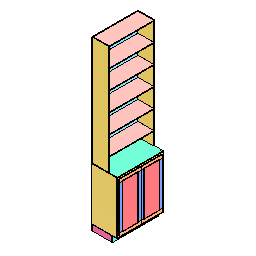
MS_BookShelves (Autodesk Fusion 360 design; units mm, degrees)
Autodesk Fusion 360 part; units mm, degrees
sketch "Part List" plane through (0, 0, 0) normal (1, 0, 0) x (0, 1, 0)
  line L0 (-117.4604, 5.2821) -> (-27.4764, 5.2821) construction
  line L1 (-27.4764, 5.2821) -> (-27.4764, 106.5384) construction
  line L2 (-27.4764, 106.5384) -> (-117.4604, 106.5384) construction
  line L3 (-117.4604, 106.5384) -> (-117.4604, 5.2821) construction
  dimension "d1" = 2
sketch "Room" plane through (0, 0, 0) normal (0, 0, 1) x (1, 0, 0)
  line L0 (922.3375, 3178.175) -> (2225.675, 3178.175) construction
  line L1 (0, 3178.175) -> (922.3375, 3178.175) construction
  line L2 (2225.675, 3178.175) -> (3114.675, 3178.175) construction
  line L3 (2259.0125, 0) -> (1363.6625, 0) construction
  line L4 (1363.6625, 46.449) -> (2259.0125, 46.449) construction
  line L5 (3114.675, 3178.175) -> (3630.6125, 3178.175) construction
  line L6 (0, 0) -> (0, 3178.175) construction
  line L7 (1363.6625, 0) -> (1363.6625, 46.449) construction
  line L8 (58.5758, 2317.75) -> (0, 2317.75) construction
  line L9 (0, 2403.475) -> (58.5758, 2403.475) construction
  line L10 (58.5758, 2403.475) -> (58.5758, 2317.75) construction
  line L11 (140.5097, 3178.175) -> (140.5097, 2420.9375) construction
  line L12 (0, 2317.75) -> (0, 2403.475) construction
  line L13 (0, 0) -> (3648.075, 0) construction
  line L14 (2259.0125, 46.449) -> (2259.0125, 0) construction
  point P0 (0, 2403.475)
  point P1 (0, 2317.75)
  point P2 (2259.0125, 0)
  point P3 (1363.6625, 0)
  dimension "d2" = 3648.075
  dimension "d3" = 895.35
  dimension "d4" = 1363.6625
  dimension "d5" = 1389.0625
  dimension "d6" = 3178.175
  dimension "d7" = 922.3375
  dimension "d8" = 1303.3375
  dimension "d9" = 889
  dimension "d10" = 515.9375
  dimension "d11" = 3630.6125
  dimension "d12" = 774.7
  dimension "d13" = 85.725
  dimension "d14" = 757.2375
  dimension "d15" = 90
  constraint coincident L6.start L13.start
  constraint horizontal L13
  constraint coincident P3 L13
  constraint coincident P2 L13
  constraint horizontal L3
  constraint vertical L7
  constraint horizontal L4
  constraint vertical L14
  constraint coincident P2 L3.start
  constraint perpendicular L6 L13
  constraint perpendicular L1 L6
  constraint parallel L0 L1
  constraint parallel L0 L2
  constraint parallel L2 L5
  constraint coincident P0 L6
  constraint coincident P1 L6
  constraint horizontal L9
  constraint vertical L10
  constraint horizontal L8
  constraint vertical L12
  constraint coincident P0 L9.start
  constraint coincident L11.start L1
  constraint perpendicular L1 L11
  measures "d2" distance of L13.end L6.start
  measures "d3" distance of P2 P3
  measures "d4" distance of L6.start P3
  measures "d5" distance of L13.end P2
  measures "d6" distance of L6.start L1.start
  measures "d7" distance of L1.start L0.start
  measures "d8" distance of L0.start L0.end
  measures "d9" distance of L0.end L2.end
  measures "d10" distance of L2.end L5.end
  measures "d11" distance of L1.start L5.end
  measures "d12" distance of L1.start P0
  measures "d13" distance of P0 P1
  measures "d14" distance of L11.start L11.end
  measures "d15" angle of L1 L11
sketch "Celing" plane through (0, 0, 0) normal (0, 0, 1) x (1, 0, 0)
  line L0 (0, 0, 2743.2) -> (3648.075, 0, 2743.2)
  line L1 (3648.075, 0, 2743.2) -> (3648.075, 3178.175, 2743.2)
  line L2 (3648.075, 3178.175, 2743.2) -> (0, 3178.175, 2743.2)
  line L3 (0, 3178.175, 2743.2) -> (0, 0, 2743.2)
  dimension "height" = 2743.2
  dimension "width" = 3648.075
  dimension "length" = 3178.175
ref_plane "WorkPlane1" through (0, 0, 0) normal (0, 1, 0) x (0, 0, 1) in component ">>WSSi_Sides"
sketch "Sketch1" plane through (0, 0, 0) normal (0, 1, 0) x (1, 0, 0) in component ">>WSSi_Sides"
  line L0 (6.35, 0) -> (266.7, 0)
  line L1 (266.7, 0) -> (266.7, -1739.9)
  line L2 (266.7, -1739.9) -> (6.35, -1739.9)
  line L3 (6.35, -1739.9) -> (6.35, 0)
  point P0 (6.35, 0)
  dimension "Y_WSSi_Sides_Orig" = 0
  dimension "X_WSSi_Sides_Orig" = 6.35
  dimension "WSSi_Sides_Width" = 260.35
  dimension "WSSi_Sides_Length" = 1739.9
  constraint horizontal L0
  constraint vertical L1
  constraint horizontal L2
  constraint vertical L3
  constraint coincident P0 L0.start
  measures "Y_WSSi_Sides_Orig" vertical distance of origin L0.start
  measures "X_WSSi_Sides_Orig" horizontal distance of origin L0.start
  measures "WSSi_Sides_Width" distance of P0 L0.end
  measures "WSSi_Sides_Length" distance of P0 L2.end
extrude "Extrude1" add sketch "Sketch1" along normal blind 12.7 makes body 1 in component ">>WSSi_Sides"
pattern_linear "00000000-0000-0000-0000-000000000000" [suppressed] in component "~~~>WS - Sides"
ref_plane "WorkPlane1" through (0, 0, 0) normal (1, 0, 0) x (0, 1, 0) in component ">WS - Back"
sketch "Sketch1 (2)" plane through (0, 0, 0) normal (1, 0, 0) x (0, 1, 0) in component ">WS - Back"
  line L0 (0, 0) -> (736.6, 0)
  line L1 (736.6, 0) -> (736.6, 1739.9)
  line L2 (736.6, 1739.9) -> (0, 1739.9)
  line L3 (0, 1739.9) -> (0, 0)
  line L4 (12.7, 0) -> (723.9, 0)
  line L5 (723.9, 0) -> (723.9, 1727.2)
  line L6 (723.9, 1727.2) -> (12.7, 1727.2)
  line L7 (12.7, 1727.2) -> (12.7, 0)
  point P0 (12.7, 0)
  dimension "WS_Back_Width" = 736.6
  dimension "WS_Back_Length" = 1739.9
  dimension "Y_WS_Back_Orig" = 0
  dimension "X_WS_Back_Orig" = 0
  dimension "WS_Back_Rabbit_Width" = 12.7
  dimension "WS_Back_NoRabbitWidth" = 711.2
  dimension "WS_Back_NoRabbit_Length" = 1727.2
  constraint horizontal L0
  constraint vertical L1
  constraint horizontal L2
  constraint vertical L3
  constraint coincident L0 P0
  constraint horizontal L4
  constraint vertical L5
  constraint horizontal L6
  constraint vertical L7
  constraint coincident P0 L4.start
  measures "WS_Back_Width" distance of L0.start L0.end
  measures "WS_Back_Length" distance of L0.start L2.end
  measures "Y_WS_Back_Orig" vertical distance of L0.start L3.end
  measures "X_WS_Back_Orig" horizontal distance of L0.start L3.end
  measures "WS_Back_Rabbit_Width" distance of L0.start L4.start
  measures "WS_Back_NoRabbitWidth" distance of P0 L4.end
  measures "WS_Back_NoRabbit_Length" distance of P0 L6.end
extrude "Extrude1'" add sketch "Sketch1 (2)" along normal blind 12.7 separate body contours L0 L4 L5 L6 L7 makes body 2 in component ">WS - Back"
extrude "Extrude2" add sketch "Sketch1 (2)" along normal blind 6.35 contours L0 L1 L2 L3 L5 L6 L7 bodies 2 in component ">WS - Back"
ref_plane "WorkPlane1" through (12.7, 0, 0) normal (1, 0, 0) x (0, 1, 0) in component "WSS_Shelves_"
sketch "Sketch1 (3)" plane through (12.7, 0, 0) normal (1, 0, 0) x (0, 1, 0) in component "WSS_Shelves_"
  line L0 (12.7, 1727.2) -> (723.9, 1727.2)
  line L1 (12.7, 1739.9) -> (12.7, 1727.2)
  line L2 (723.9, 1739.9) -> (12.7, 1739.9)
  line L3 (723.9, 1727.2) -> (723.9, 1739.9)
  point P0 (12.7, 1727.2)
  dimension "WSS_Shelves_Length" = 711.2
  dimension "WSS_Shelves_Thickness" = 12.7
  dimension "Y_WSS_Shelves_Orig" = 12.7
  dimension "Z_WSS_Shelves_Orig" = 1727.2
  constraint horizontal L0
  constraint vertical L3
  constraint horizontal L2
  constraint vertical L1
  constraint coincident P0 L0.start
  measures "WSS_Shelves_Length" distance of P0 L0.end
  measures "WSS_Shelves_Thickness" distance of P0 L1.start
  measures "Y_WSS_Shelves_Orig" horizontal distance of origin P0
  measures "Z_WSS_Shelves_Orig" vertical distance of origin P0
extrude "Extrude1''" add sketch "Sketch1 (3)" along normal blind 254 separate body makes body 3 in component "WSS_Shelves_"
pattern_linear "00000000-0000-0000-0000-000000000000'" [suppressed] in component "~~~>WS - Shelves"
ref_plane "WorkPlane1" through (266.7, 0, 0) normal (1, 0, 0) x (0, 1, 0) in component "~~~>WS - Molding"
sketch "Sketch1 (4)" plane through (266.7, 0, 0) normal (1, 0, 0) x (0, 1, 0) in component "WSM_Molding"
  line L0 (0, 0) -> (38.1, 0)
  line L1 (38.1, 0) -> (38.1, 1739.9)
  line L2 (38.1, 1739.9) -> (0, 1739.9)
  line L3 (0, 1739.9) -> (0, 0)
  dimension "X_WSM_Molding_Orig" = 0
  dimension "Y_WSM_Molding_Orig" = 0
  dimension "WSM_Molding_Width" = 38.1
  dimension "WSM_Molding_Length" = 1739.9
  constraint horizontal L0
  constraint vertical L1
  constraint horizontal L2
  constraint vertical L3
  constraint coincident L0.start L3.end
  measures "X_WSM_Molding_Orig" horizontal distance of L0.start L3.end
  measures "Y_WSM_Molding_Orig" vertical distance of L0.start L3.end
  measures "WSM_Molding_Width" distance of L0.start L0.end
  measures "WSM_Molding_Length" distance of L0.start L2.end
extrude "Extrude1'''" add sketch "Sketch1 (4)" along normal blind 12.7 separate body makes body 4 in component "WSM_Molding"
pattern_linear "00000000-0000-0000-0000-000000000000''" [suppressed] in component "~~~>WS - Molding"
ref_plane "WorkPlane1" through (0, 0, -12.7) normal (0, 0, 1) x (1, 0, 0) in component ">>WCT_TableTop"
sketch "Sketch1 (5)" plane through (0, 0, -12.7) normal (0, 0, 1) x (1, 0, 0) in component ">>WCT_TableTop"
  line L0 (0, 0) -> (406.4, 0)
  line L1 (406.4, 0) -> (406.4, 736.6)
  line L2 (406.4, 736.6) -> (0, 736.6)
  line L3 (0, 736.6) -> (0, 0)
  dimension "Y_WC_TableTop_Orig" = 0
  dimension "X_WC_TableTop_Orig" = 0
  dimension "WCT_TableTop_Width" = 406.4
  dimension "WCT_TableTop_Length" = 736.6
  constraint horizontal L0
  constraint vertical L1
  constraint horizontal L2
  constraint vertical L3
  constraint coincident L0.start L3.end
  measures "Y_WC_TableTop_Orig" horizontal distance of L0.start L3.end
  measures "X_WC_TableTop_Orig" vertical distance of L0.start L3.end
  measures "WCT_TableTop_Width" distance of L0.start L0.end
  measures "WCT_TableTop_Length" distance of L0.start L2.end
extrude "Extrude1''''" add sketch "Sketch1 (5)" along normal blind 12.7 separate body makes body 5 in component ">>WCT_TableTop"
ref_plane "WorkPlane1" through (0, 0, -850.9) normal (0, 0, 1) x (1, 0, 0) in component ">>WCB_Bottom"
sketch "Sketch1 (6)" plane through (0, 0, -850.9) normal (0, 0, 1) x (1, 0, 0) in component ">>WCB_Bottom"
  line L0 (0, 0) -> (406.4, 0)
  line L1 (406.4, 0) -> (406.4, 736.6)
  line L2 (406.4, 736.6) -> (0, 736.6)
  line L3 (0, 736.6) -> (0, 0)
  line L4 (393.7, 12.7) -> (393.7, 723.9)
  line L5 (393.7, 723.9) -> (12.7, 723.9)
  line L6 (12.7, 723.9) -> (12.7, 12.7)
  line L7 (12.7, 12.7) -> (393.7, 12.7)
  dimension "Y_WC_Bottom_Orig" = 0
  dimension "X_WC_Bottom_Orig" = 0
  dimension "WCBo_Bottom_Width" = 406.4
  dimension "WCBo_Bottom_Length" = 736.6
  constraint horizontal L0
  constraint vertical L1
  constraint horizontal L2
  constraint vertical L3
  constraint coincident L0.start L3.end
  measures "Y_WC_Bottom_Orig" vertical distance of L0.start L3.end
  measures "X_WC_Bottom_Orig" horizontal distance of L0.start L3.end
  measures "WCBo_Bottom_Width" distance of L0.start L0.end
  measures "WCBo_Bottom_Length" distance of L0.start L2.end
extrude "Extrude1'''''" add sketch "Sketch1 (6)" along normal blind 12.7 separate body contours L4 L5 L6 L7 makes body 6 in component ">>WCB_Bottom"
extrude "Extrude2'" add sketch "Sketch1 (6)" along normal blind 6.35 bodies 6 in component ">>WCB_Bottom"
ref_plane "WorkPlane1" through (0, 0, 0) normal (0, 1, 0) x (0, 0, 1) in component ">>WCS_Sides"
sketch "Sketch1 (7)" plane through (0, 0, 0) normal (0, 1, 0) x (1, 0, 0) in component ">>WCS_Sides"
  line L0 (0, 844.55) -> (393.7, 844.55)
  line L1 (393.7, 844.55) -> (393.7, 12.7)
  line L2 (393.7, 12.7) -> (0, 12.7)
  line L3 (0, 12.7) -> (0, 844.55)
  point P0 (0, 844.55)
  dimension "X_WC_Sides_Orig" = 0
  dimension "WCS_Sides_Width" = 393.7
  dimension "WCS_Sides_Length" = 831.85
  constraint horizontal L0
  constraint vertical L1
  constraint horizontal L2
  constraint vertical L3
  constraint coincident P0 L0.start
  measures "X_WC_Sides_Orig" horizontal distance of origin L0.start
  measures "WCS_Sides_Width" distance of P0 L0.end
  measures "WCS_Sides_Length" distance of P0 L2.end
extrude "Extrude1''''''" add sketch "Sketch1 (7)" along normal blind 12.7 separate body makes body 7 in component ">>WCS_Sides"
pattern_linear "00000000-0000-0000-0000-000000000000'''" [suppressed] in component "~~~>WC - Sides"
ref_plane "WorkPlane1" through (0, 0, 0) normal (1, 0, 0) x (0, 1, 0) in component ">>WCBa_Back"
sketch "Sketch1 (8)" plane through (0, 0, 0) normal (1, 0, 0) x (0, 1, 0) in component ">>WCBa_Back"
  line L0 (12.7, -844.55) -> (723.9, -844.55)
  line L1 (723.9, -844.55) -> (723.9, -12.7)
  line L2 (723.9, -12.7) -> (12.7, -12.7)
  line L3 (12.7, -12.7) -> (12.7, -844.55)
  point P0 (12.7, -844.55)
  dimension "Y_WC_Back_Orig" = 12.7
  dimension "WCBa_Back_Width" = 711.2
  dimension "WCBa_Back_Length" = 831.85
  constraint horizontal L0
  constraint vertical L1
  constraint horizontal L2
  constraint vertical L3
  constraint coincident P0 L0.start
  measures "Y_WC_Back_Orig" horizontal distance of origin L0.start
  measures "WCBa_Back_Width" distance of P0 L0.end
  measures "WCBa_Back_Length" distance of P0 L2.end
extrude "Extrude1'''''''" add sketch "Sketch1 (8)" along normal blind 12.7 separate body makes body 8 in component ">>WCBa_Back"
ref_plane "WorkPlane1" through (0, 0, -419.1) normal (0, 0, 1) x (1, 0, 0) in component "WCS_Shelves"
sketch "Sketch1 (9)" plane through (0, 0, -419.1) normal (0, 0, 1) x (1, 0, 0) in component "WCS_Shelves"
  line L0 (12.7, 12.7) -> (393.7, 12.7)
  line L1 (393.7, 12.7) -> (393.7, 723.9)
  line L2 (393.7, 723.9) -> (12.7, 723.9)
  line L3 (12.7, 723.9) -> (12.7, 12.7)
  point P0 (12.7, 12.7)
  dimension "Y_WC_Shelves_Orig" = 12.7
  dimension "X_WC_Shelves_Orig" = 12.7
  dimension "WCS_Shelves_Width" = 381
  dimension "WCS_Shelves_Length" = 711.2
  constraint horizontal L0
  constraint vertical L1
  constraint horizontal L2
  constraint vertical L3
  constraint coincident P0 L0.start
  measures "Y_WC_Shelves_Orig" vertical distance of origin L0.start
  measures "X_WC_Shelves_Orig" horizontal distance of origin L0.start
  measures "WCS_Shelves_Width" distance of P0 L0.end
  measures "WCS_Shelves_Length" distance of P0 L2.end
extrude "Extrude1''''''''" add sketch "Sketch1 (9)" along normal blind 12.7 separate body makes body 9 in component "WCS_Shelves"
ref_plane "WorkPlane1" through (393.7, 0, 0) normal (1, 0, 0) x (0, 1, 0) in component ">>WCF - Top/Bottom"
sketch "Sketch1 (10)" plane through (393.7, 0, 0) normal (1, 0, 0) x (0, 1, 0) in component ">>WCF - Top/Bottom"
  line L0 (0, -12.7) -> (736.6, -12.7)
  line L1 (736.6, -12.7) -> (736.6, -50.8)
  line L2 (736.6, -50.8) -> (0, -50.8)
  line L3 (0, -50.8) -> (0, -12.7)
  point P0 (0, -12.7)
  dimension "Y_WCF_TopBottom_Orig" = 0
  dimension "Z_WCF_TopBottom_Orig" = 12.7
  dimension "WCF_TopBottom_Length" = 736.6
  dimension "WCF_TopBottom_Width" = 38.1
  constraint horizontal L0
  constraint vertical L1
  constraint horizontal L2
  constraint vertical L3
  constraint coincident P0 L0.start
  measures "Y_WCF_TopBottom_Orig" horizontal distance of origin L0.start
  measures "Z_WCF_TopBottom_Orig" vertical distance of origin L0.start
  measures "WCF_TopBottom_Length" distance of P0 L0.end
  measures "WCF_TopBottom_Width" distance of P0 L2.end
extrude "Extrude1'''''''''" add sketch "Sketch1 (10)" along normal blind 12.7 separate body makes body 10 in component ">>WCF - Top/Bottom"
pattern_linear "00000000-0000-0000-0000-000000000000''''" [suppressed] in component "~~~>WC - Front"
ref_plane "WorkPlane1" through (393.7, 0, 0) normal (1, 0, 0) x (0, 1, 0) in component ">>WCF - Left/Right"
sketch "Sketch1 (11)" plane through (393.7, 0, 0) normal (1, 0, 0) x (0, 1, 0) in component ">>WCF - Left/Right"
  line L0 (0, -50.8) -> (38.1, -50.8)
  line L1 (38.1, -50.8) -> (38.1, -806.45)
  line L2 (38.1, -806.45) -> (0, -806.45)
  line L3 (0, -806.45) -> (0, -50.8)
  point P0 (0, -50.8)
  dimension "Y_WCF_LeftRight_Orig" = 0
  dimension "Z_WCF_LeftRight_Orig" = 50.8
  dimension "WCF_LeftRight_Width" = 38.1
  dimension "WCF_LeftRight_Length" = 755.65
  constraint horizontal L0
  constraint vertical L1
  constraint horizontal L2
  constraint vertical L3
  constraint coincident P0 L0.start
  measures "Y_WCF_LeftRight_Orig" horizontal distance of origin L0.start
  measures "Z_WCF_LeftRight_Orig" vertical distance of origin L0.start
  measures "WCF_LeftRight_Width" distance of P0 L0.end
  measures "WCF_LeftRight_Length" distance of P0 L2.end
extrude "Extrude1''''''''''" add sketch "Sketch1 (11)" along normal blind 12.7 separate body makes body 11 in component ">>WCF - Left/Right"
pattern_linear "00000000-0000-0000-0000-000000000000'''''" [suppressed] in component "~~~>WC - Front"
ref_plane "WorkPlane1" through (406.4, 0, 0) normal (1, 0, 0) x (0, 1, 0) in component ">>WCD - Top/Bottom"
sketch "Sketch1 (12)" plane through (406.4, 0, 0) normal (1, 0, 0) x (0, 1, 0) in component ">>WCD - Top/Bottom"
  line L0 (25.4, -31.75) -> (366.7125, -31.75)
  line L1 (366.7125, -31.75) -> (366.7125, -82.55)
  line L2 (366.7125, -82.55) -> (25.4, -82.55)
  line L3 (25.4, -82.55) -> (25.4, -31.75)
  point P0 (25.4, -31.75)
  dimension "Y_WCD_TopBottom_Orig" = 25.4
  dimension "Z_WCD_TopBottom_Orig" = 31.75
  dimension "WCD_TopBottom_Length" = 341.3125
  dimension "WCD_TopBottom_Width" = 50.8
  constraint horizontal L0
  constraint vertical L1
  constraint horizontal L2
  constraint vertical L3
  constraint coincident P0 L0.start
  measures "Y_WCD_TopBottom_Orig" horizontal distance of origin L0.start
  measures "Z_WCD_TopBottom_Orig" vertical distance of origin L0.start
  measures "WCD_TopBottom_Length" distance of P0 L0.end
  measures "WCD_TopBottom_Width" distance of P0 L2.end
extrude "Extrude1'''''''''''" add sketch "Sketch1 (12)" along normal blind 12.7 separate body makes body 12 in component ">>WCD - Top/Bottom"
pattern_linear "00000000-0000-0000-0000-000000000000''''''" [suppressed] in component "~~~>WC - Doors"
ref_plane "WorkPlane1" through (406.4, 0, 0) normal (1, 0, 0) x (0, 1, 0) in component ">>WCD - Left/Right"
sketch "Sketch1 (13)" plane through (406.4, 0, 0) normal (1, 0, 0) x (0, 1, 0) in component ">>WCD - Left/Right"
  line L0 (25.4, -82.55) -> (76.2, -82.55)
  line L1 (76.2, -82.55) -> (76.2, -774.7)
  line L2 (76.2, -774.7) -> (25.4, -774.7)
  line L3 (25.4, -774.7) -> (25.4, -82.55)
  point P0 (25.4, -82.55)
  dimension "Y_WCD_LeftRight_Orig" = 25.4
  dimension "Z_WCD_LeftRight_Orig" = -82.55
  dimension "WCD_LeftRight_Width" = 50.8
  dimension "WCD_LeftRight_Length" = 692.15
  constraint horizontal L0
  constraint vertical L1
  constraint horizontal L2
  constraint vertical L3
  constraint coincident P0 L0.start
  measures "Y_WCD_LeftRight_Orig" horizontal distance of origin L0.start
  measures "Z_WCD_LeftRight_Orig" vertical distance of origin L0.start
  measures "WCD_LeftRight_Width" distance of P0 L0.end
  measures "WCD_LeftRight_Length" distance of P0 L2.end
extrude "Extrude1''''''''''''" add sketch "Sketch1 (13)" along normal blind 12.7 separate body makes body 13 in component ">>WCD - Left/Right"
pattern_linear "00000000-0000-0000-0000-000000000000'''''''" [suppressed] in component "~~~>WC - Doors"
ref_plane "WorkPlane1" through (412.75, 0, 0) normal (1, 0, 0) x (0, 1, 0) in component ">>WCD - Center"
sketch "Sketch1 (14)" plane through (412.75, 0, 0) normal (1, 0, 0) x (0, 1, 0) in component ">>WCD - Center"
  line L0 (69.85, -76.2) -> (322.2625, -76.2)
  line L1 (322.2625, -76.2) -> (322.2625, -781.05)
  line L2 (322.2625, -781.05) -> (69.85, -781.05)
  line L3 (69.85, -781.05) -> (69.85, -76.2)
  point P0 (69.85, -76.2)
  dimension "Y_WCD_Center_Orig" = 69.85
  dimension "WCD_Center_Width" = 252.4125
  dimension "WCD_Center_Length" = 704.85
  constraint horizontal L0
  constraint vertical L1
  constraint horizontal L2
  constraint vertical L3
  constraint coincident P0 L0.start
  measures "Y_WCD_Center_Orig" horizontal distance of origin L0.start
  measures "WCD_Center_Width" distance of P0 L0.end
  measures "WCD_Center_Length" distance of P0 L2.end
extrude "Extrude1'''''''''''''" add sketch "Sketch1 (14)" along normal blind 6.35 separate body makes body 14 in component ">>WCD - Center"
pattern_linear "00000000-0000-0000-0000-000000000000''''''''" [suppressed] in component "~~~>WC - Doors"
ref_plane "WorkPlane1" through (0, 0, 0) normal (1, 0, 0) x (0, 1, 0) in component ">WTG - Front/Back"
sketch "Sketch1 (15)" plane through (0, 0, 0) normal (1, 0, 0) x (0, 1, 0) in component ">WTG - Front/Back"
  line L0 (0, -850.9) -> (736.6, -850.9)
  line L1 (736.6, -850.9) -> (736.6, -939.8)
  line L2 (736.6, -939.8) -> (0, -939.8)
  line L3 (0, -939.8) -> (0, -850.9)
  point P0 (0, -850.9)
  dimension "Z_WTG_FrontBack_Orig" = 850.9
  dimension "Y_WTG_FrontBack_Orig" = 0
  dimension "WTG_FrontBack_Length" = 736.6
  dimension "WTG_FrontBack_Width" = 88.9
  constraint horizontal L0
  constraint vertical L1
  constraint horizontal L2
  constraint vertical L3
  constraint coincident P0 L0.start
  measures "Z_WTG_FrontBack_Orig" vertical distance of origin L0.start
  measures "Y_WTG_FrontBack_Orig" horizontal distance of origin L0.start
  measures "WTG_FrontBack_Length" distance of P0 L0.end
  measures "WTG_FrontBack_Width" distance of P0 L2.end
extrude "Extrude1''''''''''''''" add sketch "Sketch1 (15)" along normal blind 12.7 separate body makes body 15 in component ">WTG - Front/Back"
pattern_linear "00000000-0000-0000-0000-000000000000'''''''''" [suppressed] in component "~~~West Toe Guard"
ref_plane "WorkPlane1" through (0, 0, 0) normal (0, 1, 0) x (0, 0, 1) in component ">WTG - Left/Right"
sketch "Sketch1 (16)" plane through (0, 0, 0) normal (0, 1, 0) x (1, 0, 0) in component ">WTG - Left/Right"
  line L0 (12.7, 850.9) -> (317.5, 850.9)
  line L1 (317.5, 850.9) -> (317.5, 939.8)
  line L2 (317.5, 939.8) -> (12.7, 939.8)
  line L3 (12.7, 939.8) -> (12.7, 850.9)
  point P0 (12.7, 850.9)
  dimension "X_WTG_LeftRight_Orig" = 12.7
  dimension "Z_WTG_LeftRight_Orig" = 850.9
  dimension "WTG_LeftRight_Length" = 304.8
  dimension "WTG_LeftRight_Width" = 88.9
  constraint horizontal L0
  constraint vertical L1
  constraint horizontal L2
  constraint vertical L3
  constraint coincident P0 L0.start
  measures "X_WTG_LeftRight_Orig" horizontal distance of origin L0.start
  measures "Z_WTG_LeftRight_Orig" vertical distance of origin L0.start
  measures "WTG_LeftRight_Length" distance of P0 L0.end
  measures "WTG_LeftRight_Width" distance of P0 L2.end
extrude "Extrude1'''''''''''''''" add sketch "Sketch1 (16)" along normal blind 12.7 separate body makes body 16 in component ">WTG - Left/Right"
pattern_linear "00000000-0000-0000-0000-000000000000''''''''''" [suppressed] in component "~~~West Toe Guard"
ref_plane "WorkPlane1" through (0, 0, -850.9) normal (0, 0, 1) x (1, 0, 0) in component ">WTG - Brace"
sketch "Sketch1 (17)" plane through (0, 0, -850.9) normal (0, 0, 1) x (1, 0, 0) in component ">WTG - Brace"
  line L0 (12.7, 120.65) -> (12.7, -116.3872) construction
  line L1 (12.7, 120.65) -> (120.4631, 12.8869)
  line L2 (12.7, 120.65) -> (354.6668, 120.65) construction
  line L3 (-14.2408, 93.7092) -> (93.5223, -14.0538)
  line L4 (120.4631, 12.8869) -> (107.0103, -0.5659) construction
  line L5 (120.4631, 12.8869) -> (-184.3369, 12.8869)
  line L6 (12.7, 120.65) -> (12.7, -184.15)
  point P0 (12.7, 120.65)
  dimension "Y_WTG_Brace_Orig" = 120.65
  dimension "X_WTG_Brace_Orig" = 12.7
  dimension "WTG_Brace_Angle" = 45
  dimension "WTG_Brace_Length" = 152.4
  dimension "WTG_Brace_Thickness" = 38.1
  dimension "d378" = 304.8
  dimension "WTG_Brace_Miters" = 45
  dimension "d380" = 304.8
  dimension "WTG_Brace_Miters1" = 45
  constraint coincident P0 L0.start
  constraint vertical L0
  constraint horizontal L2
  constraint perpendicular L1 L4
  measures "Y_WTG_Brace_Orig" vertical distance of origin L0.start
  measures "X_WTG_Brace_Orig" horizontal distance of origin L0.start
  measures "WTG_Brace_Angle" angle of L1 L2
  measures "WTG_Brace_Length" distance of P0 L1.end
  measures "d378" distance of L1.end L5.end
  measures "WTG_Brace_Miters" angle of L4 L5
  measures "d380" distance of P0 L6.end
  measures "WTG_Brace_Miters1" angle of L1 L6
extrude "Extrude1''''''''''''''''" add sketch "Sketch1 (17)" against normal blind 88.9 separate body contours L1 L3 L5 L6 makes body 17 in component ">WTG - Brace"
pattern_linear "00000000-0000-0000-0000-000000000000'''''''''''" [suppressed] in component "~~~West Toe Guard"
pattern_linear "00000000-0000-0000-0000-000000000000''''''''''''" [suppressed] in component "~~~West Toe Guard"
component "~~~West Shelves" placed x (1, 0, 0) y (0, 1, 0) z (0, 0, 1) at (0, 0, 0)
component "~~~West Cabinet" placed x (1, 0, 0) y (0, 1, 0) z (0, 0, 1) at (0, 0, 0)
component "~~~West Toe Guard" placed x (1, 0, 0) y (0, 1, 0) z (0, 0, 1) at (0, 0, 0)
component "North Shelves" placed x (1, 0, 0) y (0, 1, 0) z (0, 0, 1) at (0, 0, 0)
component "North Cabinet" placed x (1, 0, 0) y (0, 1, 0) z (0, 0, 1) at (0, 0, 0)
component "North Toe Guard" placed x (1, 0, 0) y (0, 1, 0) z (0, 0, 1) at (0, 0, 0)
component "~~~>WS - Sides" placed x (1, 0, 0) y (0, 1, 0) z (0, 0, 1) at (0, 0, 0) in component "~~~West Shelves"
component ">WS - Back" placed x (1, 0, 0) y (0, 1, 0) z (0, 0, 1) at (0, 0, 0) in component "~~~West Shelves"
component "~~~>WS - Molding" placed x (1, 0, 0) y (0, 1, 0) z (0, 0, 1) at (0, 0, 0) in component "~~~West Shelves"
component "~~~>WS - Shelves" placed x (1, 0, 0) y (0, 1, 0) z (0, 0, 1) at (0, 0, 0) in component "~~~West Shelves"
component "~~~WC - Table Top" placed x (1, 0, 0) y (0, 1, 0) z (0, 0, 1) at (0, 0, 0) in component "~~~West Cabinet"
component "~~~>WC - Bottom" placed x (1, 0, 0) y (0, 1, 0) z (0, 0, 1) at (0, 0, 0) in component "~~~West Cabinet"
component "~~~>WC - Sides" placed x (1, 0, 0) y (0, 1, 0) z (0, 0, 1) at (0, 0, 0) in component "~~~West Cabinet"
component "~~~>WC - Back" placed x (1, 0, 0) y (0, 1, 0) z (0, 0, 1) at (0, 0, 0) in component "~~~West Cabinet"
component "~~~>WC - Front" placed x (1, 0, 0) y (0, 1, 0) z (0, 0, 1) at (0, 0, 0) in component "~~~West Cabinet"
component "~~~>WC - Doors" placed x (1, 0, 0) y (0, 1, 0) z (0, 0, 1) at (0, 0, 0) in component "~~~West Cabinet"
component ">WC - Molding" placed x (1, 0, 0) y (0, 1, 0) z (0, 0, 1) at (0, 0, 0) in component "~~~West Cabinet"
component "~~~>WC - Shelves" placed x (1, 0, 0) y (0, 1, 0) z (0, 0, 1) at (0, 0, 0) in component "~~~West Cabinet"
component ">WTG - Front/Back" placed x (1, 0, 0) y (0, 1, 0) z (0, 0, 1) at (0, 0, 0) in component "~~~West Toe Guard"
component ">WTG - Left/Right" placed x (1, 0, 0) y (0, 1, 0) z (0, 0, 1) at (0, 0, 0) in component "~~~West Toe Guard"
component ">WTG - Brace" placed x (1, 0, 0) y (0, 1, 0) z (0, 0, 1) at (0, 0, 0) in component "~~~West Toe Guard"
component ">WTG - Front/Back" placed x (1, 0, 0) y (0, 1, 0) z (0, 0, 1) at (317.5, 0, 0) in component "~~~West Toe Guard"
component ">WTG - Left/Right" placed x (1, 0, 0) y (0, 1, 0) z (0, 0, 1) at (0, 723.9, 0) in component "~~~West Toe Guard"
component ">WTG - Brace" placed x (0, 1, 0) y (-1, 0, 0) z (0, 0, 1) at (330.2, 0.1869, 0) in component "~~~West Toe Guard"
component ">WTG - Brace" placed x (0, -1, 0) y (1, 0, 0) z (0, 0, 1) at (-0.1869, 736.6, 0) in component "~~~West Toe Guard"
component ">WTG - Brace" placed x (-1, 0, 0) y (0, -1, 0) z (0, 0, 1) at (330.0131, 736.7869, 0) in component "~~~West Toe Guard"
component ">>WSSi_Sides" placed x (1, 0, 0) y (0, 1, 0) z (0, 0, 1) at (0, 0, 0) in component "~~~>WS - Sides"
component ">>WSSi_Sides" placed x (1, 0, 0) y (0, 1, 0) z (0, 0, 1) at (0, 723.9, 0) in component "~~~>WS - Sides"
component "WSM_Molding" placed x (1, 0, 0) y (0, 1, 0) z (0, 0, 1) at (0, 0, 0) in component "~~~>WS - Molding"
component "WSM_Molding" placed x (1, 0, 0) y (0, 1, 0) z (0, 0, 1) at (0, 698.5, 0) in component "~~~>WS - Molding"
component ">>WCT_TableTop" placed x (1, 0, 0) y (0, 1, 0) z (0, 0, 1) at (0, 0, 0) in component "~~~WC - Table Top"
component ">>WCB_Bottom" placed x (1, 0, 0) y (0, 1, 0) z (0, 0, 1) at (0, 0, 0) in component "~~~>WC - Bottom"
component ">>WCS_Sides" placed x (1, 0, 0) y (0, 1, 0) z (0, 0, 1) at (0, 0, 0) in component "~~~>WC - Sides"
component ">>WCS_Sides" placed x (1, 0, 0) y (0, 1, 0) z (0, 0, 1) at (0, 723.9, 0) in component "~~~>WC - Sides"
component ">>WCBa_Back" placed x (1, 0, 0) y (0, 1, 0) z (0, 0, 1) at (0, 0, 0) in component "~~~>WC - Back"
component ">>WCF - Top/Bottom" placed x (1, 0, 0) y (0, 1, 0) z (0, 0, 1) at (0, 0, 0) in component "~~~>WC - Front"
component ">>WCF - Left/Right" placed x (1, 0, 0) y (0, 1, 0) z (0, 0, 1) at (0, 0, 0) in component "~~~>WC - Front"
component ">>WCF - Top/Bottom" placed x (1, 0, 0) y (0, 1, 0) z (0, 0, 1) at (0, 0, -793.75) in component "~~~>WC - Front"
component ">>WCF - Left/Right" placed x (1, 0, 0) y (0, 1, 0) z (0, 0, 1) at (0, 698.5, 0) in component "~~~>WC - Front"
component ">>WCD - Top/Bottom" placed x (1, 0, 0) y (0, 1, 0) z (0, 0, 1) at (0, 0, 0) in component "~~~>WC - Doors"
component ">>WCD - Left/Right" placed x (1, 0, 0) y (0, 1, 0) z (0, 0, 1) at (0, 0, 0) in component "~~~>WC - Doors"
component ">>WCD - Center" placed x (1, 0, 0) y (0, 1, 0) z (0, 0, 1) at (0, 0, 0) in component "~~~>WC - Doors"
component ">>WCD - Top/Bottom" placed x (1, 0, 0) y (0, 1, 0) z (0, 0, 1) at (0, 0, -742.95) in component "~~~>WC - Doors"
component ">>WCD - Left/Right" placed x (1, 0, 0) y (0, 1, 0) z (0, 0, 1) at (0, 290.5125, 0) in component "~~~>WC - Doors"
component ">>WCD - Top/Bottom" placed x (1, 0, 0) y (0, 1, 0) z (0, 0, 1) at (0, 344.4875, 0) in component "~~~>WC - Doors"
component ">>WCD - Left/Right" placed x (1, 0, 0) y (0, 1, 0) z (0, 0, 1) at (0, 344.4875, 0) in component "~~~>WC - Doors"
component ">>WCD - Center" placed x (1, 0, 0) y (0, 1, 0) z (0, 0, 1) at (0, 344.4875, 0) in component "~~~>WC - Doors"
component ">>WCD - Top/Bottom" placed x (1, 0, 0) y (0, 1, 0) z (0, 0, 1) at (0, 344.4875, -742.95) in component "~~~>WC - Doors"
component ">>WCD - Left/Right" placed x (1, 0, 0) y (0, 1, 0) z (0, 0, 1) at (0, 635, 0) in component "~~~>WC - Doors"
component "WCM - West Top/Bottom" placed x (1, 0, 0) y (0, 1, 0) z (0, 0, 1) at (0, 0, 0) in component ">WC - Molding"
component "WC_M - West Left/Right" placed x (1, 0, 0) y (0, 1, 0) z (0, 0, 1) at (0, 0, 0) in component ">WC - Molding"
component "WC_M - North Top/Bottom" placed x (1, 0, 0) y (0, 1, 0) z (0, 0, 1) at (0, 0, 0) in component ">WC - Molding"
component "WC_M - North Left/Right" placed x (1, 0, 0) y (0, 1, 0) z (0, 0, 1) at (0, 0, 0) in component ">WC - Molding"
component "WCS_Shelves" placed x (1, 0, 0) y (0, 1, 0) z (0, 0, 1) at (0, 0, 0) in component "~~~>WC - Shelves"
component "WSS_Shelves_" placed x (1, 0, 0) y (0, 1, 0) z (0, 0, 1) at (0, 0, 0) in component "~~~>WS - Shelves"
component "WSS_Shelves_" placed x (1, 0, 0) y (0, 1, 0) z (0, 0, 1) at (0, 0, -304.8) in component "~~~>WS - Shelves"
component "WSS_Shelves_" placed x (1, 0, 0) y (0, 1, 0) z (0, 0, 1) at (0, 0, -609.6) in component "~~~>WS - Shelves"
component "WSS_Shelves_" placed x (1, 0, 0) y (0, 1, 0) z (0, 0, 1) at (0, 0, -914.4) in component "~~~>WS - Shelves"
component "WSS_Shelves_" placed x (1, 0, 0) y (0, 1, 0) z (0, 0, 1) at (0, 0, -1219.2) in component "~~~>WS - Shelves"
component "WSS_Shelves_" placed x (1, 0, 0) y (0, 1, 0) z (0, 0, 1) at (0, 0, -1524) in component "~~~>WS - Shelves"
equation "room_W_wall = 10'-0\" + 5\" + 0.125 in"
equation "room_distance_to_ceiling = 9 ft"
equation "room_shelves_depth = 11\" + 0'- 1/16\""
equation "room_shelves_width = 5'-0\" + 0'- 9/16\""
equation "room_shelves_height = 58.75 in"
equation "room_doors_left = 2'-0\" + 5\" + 0'- 13/16\""
equation "room_doors_right = room_doors_left"
equation "room_doorframe_left = 2'-0\" + 11\""
equation "room_doorframe_right = room_doorframe_left"
equation "room_NS_wall = 11'-0\" + 10.75 in"
equation "room_S_wall_right = 4'-0\" + 5\" + 0'- 11/16\""
equation "room_S_wall_left = 4'-0\" + 6\" + 0'- 11/16\""
equation "room_S_wall_window = 2'-0\" + 11.25 in"
equation "room_S_wall_total = room_S_wall_left + room_S_wall_right + room_S_wall_window"
equation "room_N_wall_p1 = 3'-0\" + 0'- 5/16\""
equation "room_N_wall_p2 = 4'-0\" + 3\" + 0'- 5/16\""
equation "room_N_wall_p3 = 1'-0\" + 8\" + 0'- 5/16\""
equation "room_W_outlet_NWallToRight = 2'-0\" + 6.5 in"
equation "room_W_outlet_floorToBtm = 11\" + 0'- 5/8\""
equation "room_W_outlet_floorToTop = 1'-0\" + 4\" + 0'- 11/16\""
equation "room_W_outlet_NWallToLeft = 2'-0\" + 9\" + 0'- 7/8\""
equation "room_W_outlet_length = room_W_outlet_floorToTop - room_W_outlet_floorToBtm"
equation "room_W_outlet_width = room_W_outlet_NWallToLeft - room_W_outlet_NWallToRight"
equation "Shared_Material_Thickness = 0.5 in"
equation "Shared_WSS_Shelves_Width = 10 in"
equation "Shared_WestCabinet_TotalHeight = 3'-0\" - cabinet_toe_guard"
equation "Shared_W_Total_Width = room_W_wall - 36\""
equation "Shared_W_Cabinet_Depth = Shared_WSS_Shelves_Width + 6\""
equation "Shared_W_Total_Height = room_distance_to_ceiling - Shared_WestCabinet_TotalHeight - Shared_Material_Thickness - cabinet_toe_guard - 3\""
equation "cabinet_toe_guard = material_toe_width"
equation "Shared_W_NumOfSections = 3"
equation "Shared_WSS_Shelves_Length = Shared_W_Section_Width - ( Shared_WCS_Sides_Thickness * 2 )"
equation "material_toe_width = 3.0 in"
equation "material_toe_thickness = 1.5 in"
equation "toe_bracket = 6 in"
equation "Shared_WCF_Bezzle = 1.5 in"
equation "Shared_WSSi_Sides_length = Shared_W_Total_Height"
equation "shlf_W_molding_width = 1.5 in"
equation "shlf_W_molding_length = Shared_WSSi_Sides_length"
equation "shlf_W_molding_origin = 0.001 in"
equation "height = room_distance_to_ceiling"
equation "width = room_S_wall_total"
equation "length = room_W_wall"
equation "Z_WSSi_Sides_Orig = 0 ft"
equation "X_WSSi_Sides_Orig = Shared_WS_Back_Rabbit_Depth"
equation "WSSi_Sides_Width = Shared_WSSi_Sides_Width"
equation "WSSi_Sides_Length = Shared_WSSi_Sides_length"
equation "WSSi_Sides_Thickness = Shared_WSSi_Sides_Thickness"
equation "WS_Sides_NumOfSides = 2"
equation "WS_Sides_DistanceBTWSides = Shared_WS_Sides_DistanceBTWSides"
equation "Z_WS_Back_Orig = 0 in"
equation "WS_Back_Width = Shared_WS_Back_Width"
equation "WS_Back_Length = Shared_W_Total_Height"
equation "WS_Back_Thickness = Shared_WS_Back_Thickness"
equation "WS_Back_Rabbit_Depth = Shared_WS_Back_Rabbit_Depth"
equation "Shared_WS_Back_Thickness = Shared_Material_Thickness"
equation "WS_Back_Rabbit_Width = Shared_WSSi_Sides_Thickness"
equation "WS_Back_NoRabbitWidth = WS_Back_Width - ( Shared_WSS_Shelves_Thickness * 2 )"
equation "WS_Back_NoRabbit_Length = WS_Back_Length - Shared_WSS_Shelves_Thickness"
equation "X_WSS_Shelves_Orig1 = 2 in"
equation "X_WSS_Shelves_Orig = WS_Back_Thickness"
equation "Shared_WS_Sides_DistanceBTWSides = -( Shared_W_Section_Width - Shared_WSSi_Sides_Thickness )"
equation "Shared_WSS_Shelves_Thickness = 0.5 in"
equation "Shared_WSSi_Sides_Thickness = Shared_Material_Thickness"
equation "Shared_WS_Back_Rabbit_Depth = Shared_WS_Back_Thickness / 2"
equation "Z_WS_Molding_Orig = Shared_WS_Back_Rabbit_Depth + Shared_WSSi_Sides_Width"
equation "WSM_Molding_Length = Shared_WSSi_Sides_length"
equation "WSM_Molding_Thickness = Shared_WSM_Molding_Thickness"
equation "Shared_WSM_Molding_Thickness = Shared_Material_Thickness"
equation "Shared_WSSi_Sides_Width = Shared_WSS_Shelves_Width + Shared_WS_Back_Rabbit_Depth"
equation "WSM_Molding_Num = 2"
equation "WSM_Molding_SpaceBTWMolding = Shared_WS_Back_Width - WSM_Molding_Width"
equation "Shared_WS_Back_Width = Shared_WSS_Shelves_Length + ( Shared_WSSi_Sides_Thickness * 2 )"
equation "Z_WC_TableTop_Orig = -( Shared_WCT_TableTop_Thickness )"
equation "WCT_TableTop_Width = Shared_W_Cabinet_Depth"
equation "WCT_TableTop_Length = Shared_WS_Back_Width"
equation "WCT_TableTop_Thickness = Shared_WCT_TableTop_Thickness"
equation "Shared_WCT_TableTop_Thickness = Shared_Material_Thickness"
equation "Z_WC_Bottom_Orig = -( abs(Z_WC_Sides_Orig) + WCBo_Bottom_Rabbit_Depth )"
equation "WCBo_Bottom_Width = Shared_W_Cabinet_Depth"
equation "WCBo_Bottom_Length = Shared_WSS_Shelves_Length + ( Shared_WCS_Sides_Thickness * 2 )"
equation "WCBo_Bottom_Rabbit_Width = -( Shared_WCBo_Bottom_Thickness )"
equation "WCBo_Bottom_Thickness = Shared_WCBo_Bottom_Thickness"
equation "WCBo_Bottom_Rabbit_Depth = Shared_WCBo_Bottom_Thickness / 2"
equation "Shared_WCBo_Bottom_Thickness = Shared_Material_Thickness"
equation "Y_WC_Sides_Orig = 0 in"
equation "Z_WC_Sides_Orig = -( WCS_Sides_Length + Shared_WCT_TableTop_Thickness )"
equation "WCS_Sides_Width = Shared_W_Cabinet_Depth - abs(WCBo_Bottom_Rabbit_Width)"
equation "WCS_Sides_Length = Shared_WestCabinet_TotalHeight - WCBo_Bottom_Rabbit_Depth"
equation "WCS_Sides_Thickness = Shared_WCS_Sides_Thickness"
equation "Shared_WCS_Sides_Thickness = Shared_Material_Thickness"
equation "Shared_W_Section_Width = floor(Shared_W_Total_Width / Shared_W_NumOfSections)"
equation "WC_Sides_NumOfSides = 2"
equation "WC_Sides_DistBTWSides = -( Shared_W_Section_Width - WCS_Sides_Thickness )"
equation "X_WC_Back_Orig = 0 in"
equation "Z_WC_Back_Orig = -( WCBa_Back_Length + Shared_WCT_TableTop_Thickness )"
equation "Y_WC_Back_Orig = Shared_WCS_Sides_Thickness"
equation "WCBa_Back_Width = Shared_W_Section_Width - ( Shared_WCS_Sides_Thickness * 2 )"
equation "WCBa_Back_Length = Shared_WestCabinet_TotalHeight - ( Shared_Material_Thickness / 2 )"
equation "WCBa_Back_Thickness = Shared_WCBa_Back_Thickness"
equation "Shared_WCBa_Back_Thickness = Shared_Material_Thickness"
equation "Z_WC_Shelves_Orig = -( Shared_WestCabinet_TotalHeight / 2 )"
equation "Y_WC_Shelves_Orig = Shared_WCS_Sides_Thickness"
equation "X_WC_Shelves_Orig = Shared_WCBa_Back_Thickness"
equation "WCS_Shelves_Width = Shared_W_Cabinet_Depth - Shared_WCBa_Back_Thickness - abs(WCBo_Bottom_Rabbit_Width)"
equation "WCS_Shelves_Length = Shared_W_Section_Width - ( Shared_WCS_Sides_Thickness * 2 )"
equation "WCS_Shelves_Thickness = Shared_WCS_Shelves_Thickness"
equation "Shared_WCS_Shelves_Thickness = Shared_Material_Thickness"
equation "X_WCF_TopBottom_Orig = Shared_W_Cabinet_Depth - WCF_TopBottom_Thickness"
equation "Z_WCF_TopBottom_Orig = Shared_WCT_TableTop_Thickness"
equation "WCF_TopBottom_Length = Shared_W_Section_Width"
equation "WCF_TopBottom_Width = Shared_WCF_Bezzle"
equation "WCF_TopBottom_Thickness = Shared_Material_Thickness"
equation "WCF_TopBottom_Num = 2"
equation "WCF_TopBottom_DistBTWFronts = -( Shared_WestCabinet_TotalHeight - WCF_TopBottom_Width - ( Shared_WCBo_Bottom_Thickness - WCBo_Bottom_Rabbit_Depth ) )"
equation "X_WCF_LeftRight_Orig = Shared_W_Cabinet_Depth - Shared_WS_Back_Thickness"
equation "Z_WCF_LeftRight_Orig = WCT_TableTop_Thickness + WCF_TopBottom_Width"
equation "WCF_LeftRight_Width = Shared_WCF_Bezzle"
equation "WCF_LeftRight_Length = Shared_WestCabinet_TotalHeight - ( WCF_TopBottom_Width * 2 ) - WCBo_Bottom_Rabbit_Depth"
equation "WCF_LeftRight_Thickness = Shared_Material_Thickness"
equation "WCF_LeftRight_Num = 2"
equation "WCF_LeftRight_DistBTWFronts = Shared_W_Section_Width - WCF_LeftRight_Width"
equation "X_WCD_TopBottom = Shared_W_Cabinet_Depth"
equation "Y_WCD_TopBottom_Orig = WCF_LeftRight_Width - Shared_WCD_OverlayOffset"
equation "Z_WCD_TopBottom_Orig = WCT_TableTop_Thickness + WCF_TopBottom_Width - ( WCF_LeftRight_Width / 2 )"
equation "WCD_TopBottom_Length = ( Shared_W_Section_Width / 2 ) - Y_WCD_LeftRight_Orig - ( Shared_WCD_GapBTWDoors / 2 )"
equation "WCD_TopBottom_Width = Shared_WCD_Bezzel"
equation "WCD_TopBottom_Thickness = Shared_WCD_TopBottom_Thickness"
equation "Shared_WCD_TopBottom_Thickness = Shared_Material_Door"
equation "d246 = -( Shared_WestCabinet_TotalHeight - WCT_TableTop_Thickness - WCD_TopBottom_Width - ( ( 0.5 * 2 ) * 1 in ) - WCBo_Bottom_Rabbit_Depth )"
equation "X_WCD_LeftRight_Orig = Shared_W_Cabinet_Depth"
equation "Y_WCD_LeftRight_Orig = Y_WCD_TopBottom_Orig"
equation "Z_WCD_LeftRight_Orig = -( WCT_TableTop_Thickness + ( WCF_TopBottom_Width / 2 ) + WCD_TopBottom_Width )"
equation "WCD_LeftRight_Width = Shared_WCD_Bezzel"
equation "WCD_LeftRight_Length = Shared_WestCabinet_TotalHeight - ( WCD_TopBottom_Width * 2 ) - WCF_TopBottom_Width - WCBo_Bottom_Rabbit_Depth"
equation "WCD_LeftRight_Thickness = Shared_WCD_LeftRight_Thickness"
equation "WCD_LeftRight_DistBTWLR = WCD_TopBottom_Length - WCD_LeftRight_Width"
equation "X_WCD_Center_Orig = X_WCD_TopBottom + Shared_WCD_Dado_Depth"
equation "Z_WCD_Center_Orig = -( Z_WCD_LeftRight_Orig + Shared_WCD_Dado_Depth )"
equation "Y_WCD_Center_Orig = Y_WCD_LeftRight_Orig + WCD_LeftRight_Width - Shared_WCD_Dado_Depth"
equation "WCD_Center_Width = WCD_TopBottom_Length - ( WCD_LeftRight_Width * 2 ) + ( Shared_WCD_Dado_Depth * 2 )"
equation "WCD_Center_Length = WCD_LeftRight_Length + ( Shared_WCD_Dado_Depth * 2 )"
equation "WCD_Center_Thickness = Shared_WCD_Center_Thickness"
equation "Shared_Material_Center = 0.25 in"
equation "Shared_WCD_LeftRight_Thickness = Shared_Material_Door"
equation "Shared_WCD_Center_Thickness = Shared_Material_Center"
equation "Shared_WCD_Dado_Depth = 0.25 in"
equation "Shared_WCD_Bezzel = 2 in"
equation "Shared_WCD_GapBTWDoors = 0.125 in"
equation "WCD_NumOfDoors = 2"
equation "WCD_DistBTWDoors = Shared_W_Section_Width - ( 2 * Y_WCD_LeftRight_Orig ) - WCD_TopBottom_Length"
equation "Shared_WCD_OverlayOffset = 0.5 in"
equation "WS_Shelves_DistBTWShelves_ = 12 in"
equation "Shared_Material_Door = Shared_Material_Thickness"
equation "X_WTG_FrontBack_Orig = 0 in"
equation "Z_WTG_FrontBack_Orig = Shared_WestCabinet_TotalHeight + Shared_WCT_TableTop_Thickness"
equation "WTG_FrontBack_Length = Shared_W_Section_Width"
equation "WTG_FrontBack_Thickness = Shared_Material_Thickness"
equation "WTG_FrontBack_Num = 2"
equation "WTG_FrontBack_DistBTWParts = -( Shared_W_Cabinet_Depth - Shared_ToeGuard_Offset - WTG_FrontBack_Thickness )"
equation "Y_WTG_LeftRight_Orig = 0 in"
equation "X_WTG_LeftRight_Orig = WTG_FrontBack_Thickness"
equation "Z_WTG_LeftRight_Orig = Shared_WestCabinet_TotalHeight + Shared_WCT_TableTop_Thickness"
equation "WTG_LeftRight_Length = Shared_W_Cabinet_Depth - Shared_ToeGuard_Offset - ( WTG_FrontBack_Thickness * 2 )"
equation "WTG_LeftRight_Width = WTG_FrontBack_Width"
equation "Shared_ToeGuard_Offset = 3 in"
equation "WTG_LeftRight_Thickness = Shared_Material_Thickness"
equation "WTG_LeftRight_Num = 2"
equation "WTG_LeftRight_DistBTWParts = Shared_W_Section_Width - WTG_LeftRight_Thickness"
equation "Z_WTG_Brace_Orig = -( Shared_WestCabinet_TotalHeight + Shared_WCT_TableTop_Thickness )"
equation "Y_WTG_Brace_Orig = WCD_LeftRight_Thickness + 4.25 in"
equation "X_WTG_Brace_Orig = WCD_TopBottom_Thickness"
equation "WTG_Brace_Thickness = material_toe_thickness"
equation "WTG_Brace_Miters = WTG_Brace_Angle"
equation "WTG_Brace_Miters1 = WTG_Brace_Angle"
equation "WTG_Brace_Width = -3.5 in"
equation "X_WTG_Brace_DistBTWParts = WTG_LeftRight_Length - 4.25 in"
equation "Y_WTG_Brace_DistBTWParts = -( Shared_W_Section_Width - ( WTG_LeftRight_Thickness * 2 ) - 4.25 in )"
equation "X_WSS_Shelves_Orig = WS_Back_Thickness"
equation "WSS_Shelves_Length = Shared_WSS_Shelves_Length"
equation "WSS_Shelves_Thickness = Shared_WSS_Shelves_Thickness"
equation "Y_WSS_Shelves_Orig = WCS_Sides_Thickness"
equation "Z_WSS_Shelves_Orig = Shared_WSSi_Sides_length - WCS_Shelves_Thickness"
equation "WSS_Shelves_Width = Shared_WSS_Shelves_Width"
equation "WS_Shelves_NumOfShelves = floor(Shared_W_Total_Height / abs(WS_Shelves_DistBTWShelves_)) + 1"
equation "WS_Shelves_DistBTWShelves = -( 12 in )"
